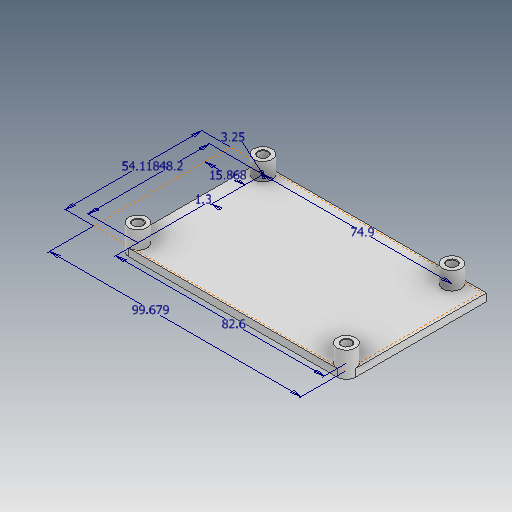
# Autodesk Inventor part: arduino_mega_standoffs_test
Saved by Autodesk Inventor 2025.1 (Build 291241000, 241)
## iProperties
Created: 2026-06-20
Part Number: arduino_mega_standoffs_test
Material: Generic
Document SubType Name: Modeling
Designer: Aiden
Density: 1 g/cm^3
Appearance: Default
Author: Aiden
Autodesk Inventor part; units mm, degrees
ref_plane "YZ Plane" through (0, 0, 0) normal (1, 0, 0) x (0, 1, 0)
ref_plane "XZ Plane" through (0, 0, 0) normal (0, 1, 0) x (-1, 0, 0)
ref_plane "XY Plane" through (0, 0, 0) normal (0, 0, 1) x (1, 0, 0)
sketch "Sketch1" plane through (0, 0, 0) normal (0, 1, 0) x (-1, 0, 0)
  circle A0 centre (43.0199, -7.0958) radius 1.625 construction
  circle A1 centre (-31.8801, -7.0958) radius 1.625 construction
  circle A2 centre (44.3199, 41.1042) radius 1.625 construction
  circle A3 centre (-38.2801, 41.1042) radius 1.625 construction
  line L0 (58.8879, -10.055) -> (-40.7911, -10.055) construction
  line L1 (-40.7911, -10.055) -> (-40.7911, 44.0634) construction
  line L2 (-40.7911, 44.0634) -> (58.8879, 44.0634) construction
  line L3 (58.8879, 44.0634) -> (58.8879, -10.055) construction
  line L4 (43.0199, -7.0958) -> (43.0199, -10.055)
  line L5 (44.3199, 41.1042) -> (44.3199, 44.0634)
  dimension "d0" = 3.25
  dimension "d1" = 74.9
  dimension "d2" = 1.3
  dimension "d3" = 48.2
  dimension "d5" = 82.6
  dimension "d9" = 15.868
  dimension "d10" = 54.1184
  dimension "d11" = 99.679
  constraints: 12 end point, 4 centre point, 3 equal radius, 3 parallel, 3 perpendicular, 2 horizontal alignment, 2 point on line, 1 horizontal
  measures "d0" diameter of A0
  measures "d1" distance of A1.centre L4.start
  measures "d2" horizontal distance of L5.start L4.start
  measures "d3" vertical distance of L4.start L5.start
  measures "d5" distance of A3.centre L5.start
  measures "d9" distance from line of L3 L4.start
  measures "d10" distance of L2.end L0.start
  measures "d11" distance of L1.end L2.end
sketch "Sketch2" plane through (0, 0, 0) normal (0, 1, 0) x (-1, 0, 0)
  circle A0 centre (43.0199, -7.0958) radius 1.625 construction
  circle A1 centre (-31.8801, -7.0958) radius 1.625 construction
  circle A2 centre (-38.2801, 41.1042) radius 1.625 construction
  circle A3 centre (44.3199, 41.1042) radius 1.625 construction
  circle A4 centre (43.0199, -7.0958) radius 3.625
  circle A5 centre (-31.8801, -7.0958) radius 3.625
  circle A6 centre (-38.2801, 41.1042) radius 3.625
  circle A7 centre (44.3199, 41.1042) radius 3.625
  point P0 (0, 0)
  dimension "d6" = 2
  constraints: 4 centre point, 4 coincident, 3 equal radius
  measures "d6" radial gap between concentric circles of A0 A4
extrude "Extrusion1" add sketch "Sketch2" along normal blind 7
sketch "Sketch3" plane through (-43.0199, 7, -7.0958) normal (0, 1, 0) x (1, 0, 0)
  circle A0 centre (0, 0) radius 3.625 projected
  circle A1 centre (74.9, 0) radius 3.625 projected
  circle A2 centre (81.3, -48.2) radius 3.625 projected
  circle A3 centre (-1.3, -48.2) radius 3.625 projected
  point P0 (43.0199, -7.0958)
  constraints: 4 coincident
hole "Hole1" at (-43.0199, 7, -7.0958) at (31.8801, 7, -7.0958) at (38.2801, 7, 41.1042) at (-44.3199, 7, 41.1042) direction (0, -1, 0) diameter 3.75 depth 4
chamfer "Chamfer1" distance 0.2 angle 45 4 edges at (-43.0199, 7, -8.9708) (31.8801, 7, -8.9708) (38.2801, 7, 39.2292) (-44.3199, 7, 39.2292)
sketch "Sketch4" plane through (-44.3199, 0, 41.1042) normal (0, -1, 0) x (1, 0, 0)
  line L0 (-3.625, 3.625) -> (86.225, 3.625)
  line L1 (86.225, 3.625) -> (86.225, -51.825)
  line L2 (86.225, -51.825) -> (-3.625, -51.825)
  line L3 (-3.625, -51.825) -> (-3.625, 3.625)
  circle A0 centre (0, 0) radius 3.625 projected
  circle A1 centre (76.2, -48.2) radius 3.625 projected
  circle A2 centre (82.6, 0) radius 3.625 projected
  point P0 (44.3199, -41.1042)
  point P1 (-3.625, 0)
  point P2 (86.225, 0)
  point P3 (82.6, 3.625)
  point P4 (0, 3.625)
  constraints: 8 end point, 4 tangent, 2 parallel, 1 horizontal, 1 perpendicular
extrude "Extrusion2" add sketch "Sketch4" along normal blind 3 contours A1 | L0 A2 L1 L2 L3 A0 | A0 | A2
body "Solid1"
